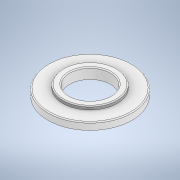
# Autodesk Inventor part: ZKE-Term-Solid-Shim
Saved by Autodesk Inventor 2021 (Build 250183000, 183)
## iProperties
Created: 2020-08-13
Part Number: ZKE-Term-Solid-Shim
Material: ABS Plastic
Document SubType Name: Modeling
Designer: lucas
Density: 1.06 g/cm^3
Appearance: Smooth - White
Project: 4Wire-Laser
Author: lucas
Revision Number: ZKE_SHIM
Autodesk Inventor part; units mm, degrees
ref_plane "YZ Plane" through (0, 0, 0) normal (1, 0, 0) x (0, 1, 0)
ref_plane "XZ Plane" through (0, 0, 0) normal (0, 1, 0) x (-1, 0, 0)
ref_plane "XY Plane" through (0, 0, 0) normal (0, 0, 1) x (1, 0, 0)
sketch "Sketch1" plane through (0, 0, 0) normal (0, 1, 0) x (-1, 0, 0)
  circle A0 centre (0, 0) radius 8.75
  circle A1 centre (0, 0) radius 5.65
  circle A2 centre (0, 0) radius 4.25
  dimension "d0" = 17.5
  dimension "d1" = 11.3
  dimension "d2" = 8.5
  constraints: 3 centre point, 3 coincident
  measures "d0" diameter of A0
  measures "d1" diameter of A1
  measures "d2" diameter of A2
extrude "Extrusion1" add sketch "Sketch1" along normal blind 2.2 contours A1
extrude "Extrusion2" add sketch "Sketch1" along normal blind 1.5 contours A0
fillet "Fillet1" radius 0.2 3 edges at (4.25, 2.2, 0) (5.65, 2.2, 0) (8.75, 1.5, 0)
body "Solid1"
